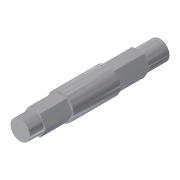
# Autodesk Inventor part: Module Live Axle
Saved by Autodesk Inventor 2014 SP1 (Build 180222100, 222)
## iProperties
Created: 2014-05-04
Part Number: Module Live Axle
Material: Aluminum 6061
Document SubType Name: Modeling
Designer: Rauhul Varma
Mass: 12.5988 g
Surface Area: 21.3062 cm^2
Volume: 4.64899 cm^3
Density: 2.71 g/cm^3
Appearance: Aluminum - Polished
Author: Rauhul Varma
Autodesk Inventor part; units mm, degrees
ref_plane "YZ Plane" through (0, 0, 0) normal (1, 0, 0) x (0, 1, 0)
ref_plane "XZ Plane" through (0, 0, 0) normal (0, 1, 0) x (-1, 0, 0)
ref_plane "XY Plane" through (0, 0, 0) normal (0, 0, 1) x (1, 0, 0)
sketch "Sketch1" plane through (0, 0, 0) normal (0, 0, 1) x (1, 0, 0)
  circle A0 centre (0, 0) radius 4.5
  dimension "d0" = 9
  constraints: 1 centre point, 1 coincident
  measures "d0" diameter of A0
extrude "Extrusion1" add sketch "Sketch1" along normal blind 9.9219
sketch "Sketch4" plane through (0, 0, 9.9219) normal (0, 0, 1) x (1, 0, 0)
  circle A0 centre (0, 0) radius 4.5 projected
  line L0 (5.4993, 0) -> (2.7496, -4.7625)
  line L1 (2.7496, -4.7625) -> (-2.7496, -4.7625)
  line L2 (-2.7496, -4.7625) -> (-5.4993, 0)
  line L3 (-5.4993, 0) -> (-2.7496, 4.7625)
  line L4 (-2.7496, 4.7625) -> (2.7496, 4.7625)
  line L5 (2.7496, 4.7625) -> (5.4993, 0)
  dimension "d9" = 9.525
  constraints: 12 end point, 1 coincident, 1 horizontal, 13 other
  measures "d9" distance between parallel lines of L1 L4
extrude "Extrusion4" add sketch "Sketch4" along normal blind 14.273 contours A0 | L0 L1 L2 L3 L4 L5
sketch "Sketch5" plane through (0, 0, 24.1949) normal (0, 0, 1) x (1, 0, 0)
  circle A0 centre (0, 0) radius 6
  dimension "d12" = 12
  constraints: 1 centre point, 1 coincident
  measures "d12" diameter of A0
extrude "Extrusion5" add sketch "Sketch5" along normal blind 21.5505
sketch "Sketch6" plane through (0, 0, 45.7454) normal (0, 0, 1) x (1, 0, 0)
  circle A0 centre (0, 0) radius 6 projected
  line L0 (5.4993, 0) -> (2.7496, -4.7625)
  line L1 (2.7496, -4.7625) -> (-2.7496, -4.7625)
  line L2 (-2.7496, -4.7625) -> (-5.4993, 0)
  line L3 (-5.4993, 0) -> (-2.7496, 4.7625)
  line L4 (-2.7496, 4.7625) -> (2.7496, 4.7625)
  line L5 (2.7496, 4.7625) -> (5.4993, 0)
  dimension "d15" = 9.525
  constraints: 12 end point, 1 coincident, 1 horizontal, 13 other
  measures "d15" distance between parallel lines of L1 L4
extrude "Extrusion6" add sketch "Sketch6" along normal blind 12.3571 contours L0 L1 L2 L3 L4 L5
sketch "Sketch7" plane through (0, 0, 58.1025) normal (0, 0, 1) x (1, 0, 0)
  circle A0 centre (0, 0) radius 4.5
  dimension "d18" = 9
  constraints: 1 centre point, 1 coincident
  measures "d18" diameter of A0
extrude "Extrusion7" add sketch "Sketch7" along normal blind 6.35
body "Solid1"
